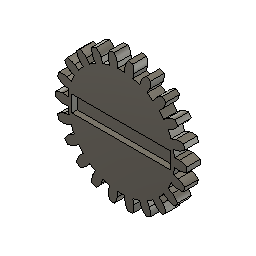
heat_controller (Autodesk Fusion 360 archive; units mm, degrees)
design "gear"
Autodesk Fusion 360 part; units mm, degrees
(part 1 of 8)
sketch "Sketch1" plane through (0, 0, 0) normal (0, 0, 1) x (1, 0, 0) in component "Component"
  spline S0 degree 5 poles (21.2374, -1.6373) (21.2376, -1.6373) (21.2379, -1.6374) (21.2384, -1.6374) (21.2392, -1.6374) (21.2403, -1.6375) (21.2417, -1.6376) (21.2433, -1.6377) (21.245, -1.6378) (21.2469, -1.6378) (21.249, -1.6379) (21.2512, -1.638) (21.2537, -1.6381) (21.2562, -1.6382) (21.259, -1.6383) (21.2619, -1.6384) (21.265, -1.6385) (21.2682, -1.6385) (21.2715, -1.6386) (21.2751, -1.6387) (21.2787, -1.6387) (21.2825, -1.6388) (21.2865, -1.6388) (21.2906, -1.6388) (21.2948, -1.6389) (21.2991, -1.6389) (21.3036, -1.6389) (21.3083, -1.6388) (21.313, -1.6388) (21.3179, -1.6388) (21.3229, -1.6387) (21.3281, -1.6386) (21.3334, -1.6385) (21.3387, -1.6384) (21.3443, -1.6383) (21.3499, -1.6382) (21.3556, -1.638) (21.3615, -1.6378) (21.3675, -1.6376) (21.3736, -1.6374) (21.3798, -1.6372) (21.3861, -1.6369) (21.3925, -1.6367) (21.399, -1.6364) (21.4057, -1.636) (21.4124, -1.6357) (21.4193, -1.6353) (21.4262, -1.6349) (21.4333, -1.6345) (21.4405, -1.6341) (21.4477, -1.6336) (21.4551, -1.6332) (21.4625, -1.6327) (21.4701, -1.6321) (21.4778, -1.6316) (21.4855, -1.631) (21.4934, -1.6304) (21.5013, -1.6298) (21.5093, -1.6291) (21.5174, -1.6284) (21.5257, -1.6277) (21.534, -1.6269) (21.5423, -1.6262) (21.5508, -1.6254) (21.5594, -1.6245) (21.568, -1.6237) (21.5768, -1.6228) (21.5856, -1.6219) (21.5945, -1.621) (21.6035, -1.62) (21.6126, -1.619) (21.6217, -1.6179) (21.631, -1.6169) (21.6403, -1.6158) (21.6497, -1.6147) (21.6592, -1.6135) (21.6687, -1.6123) (21.6783, -1.6111) (21.688, -1.6098) (21.6978, -1.6086) (21.7077, -1.6072) (21.7176, -1.6059) (21.7276, -1.6045) (21.7377, -1.6031) (21.7479, -1.6017) (21.7581, -1.6002) (21.7684, -1.5987) (21.7788, -1.5971) (21.7892, -1.5955) (21.7997, -1.5939) (21.8103, -1.5923) (21.821, -1.5906) (21.8317, -1.5889) (21.8425, -1.5871) (21.8533, -1.5853) (21.8642, -1.5835) (21.8752, -1.5816) (21.8863, -1.5797) (21.8974, -1.5778) (21.9086, -1.5758) (21.9198, -1.5738) (21.9311, -1.5718) (21.9425, -1.5697) (21.9539, -1.5676) (21.9654, -1.5655) (21.977, -1.5633) (21.9886, -1.5611) (22.0003, -1.5588) (22.012, -1.5565) (22.0238, -1.5542) (22.0357, -1.5518) (22.0476, -1.5494) (22.0596, -1.547) (22.0716, -1.5445) (22.0837, -1.542) (22.0958, -1.5394) (22.108, -1.5368) (22.1203, -1.5342) (22.1326, -1.5315) (22.145, -1.5288) (22.1574, -1.5261) (22.1699, -1.5233) (22.1824, -1.5205) (22.195, -1.5176) (22.2077, -1.5147) (22.2204, -1.5118) (22.2331, -1.5088) (22.2459, -1.5058) (22.2588, -1.5027) (22.2717, -1.4996) (22.2846, -1.4965) (22.2976, -1.4933) (22.3107, -1.4901) (22.3238, -1.4868) (22.3369, -1.4835) (22.3501, -1.4802) (22.3634, -1.4768) (22.3767, -1.4734) (22.39, -1.4699) (22.4034, -1.4664) (22.4169, -1.4629) (22.4304, -1.4593) (22.4439, -1.4557) (22.4575, -1.452) (22.4711, -1.4483) (22.4848, -1.4446) (22.4985, -1.4408) (22.5123, -1.437) (22.5261, -1.4331) (22.5399, -1.4292) (22.5538, -1.4253) (22.5678, -1.4213) (22.5818, -1.4172) (22.5958, -1.4132) (22.6099, -1.4091) (22.624, -1.4049) (22.6381, -1.4007) (22.6523, -1.3965) (22.6666, -1.3922) (22.6809, -1.3879) (22.6952, -1.3835) (22.7095, -1.3791) (22.7239, -1.3747) (22.7384, -1.3702) (22.7529, -1.3656) (22.7674, -1.3611) (22.7819, -1.3564) (22.7965, -1.3518) (22.8112, -1.3471) (22.8259, -1.3423) (22.8406, -1.3376) (22.8553, -1.3327) (22.8701, -1.3279) (22.8849, -1.3229) (22.8998, -1.318) (22.9147, -1.313) (22.9297, -1.3079) (22.9446, -1.3029) (22.9596, -1.2977) (22.9747, -1.2926) (22.9898, -1.2874) (23.0049, -1.2821) (23.02, -1.2768) (23.0352, -1.2715) (23.0504, -1.2661) (23.0657, -1.2606) (23.081, -1.2552) (23.0963, -1.2496) (23.1116, -1.2441) (23.127, -1.2385) (23.1425, -1.2328) (23.1579, -1.2271) (23.1734, -1.2214) (23.1889, -1.2156) (23.2045, -1.2098) (23.22, -1.204) (23.2356, -1.198) (23.2513, -1.1921) (23.267, -1.1861) (23.2827, -1.1801) (23.2984, -1.174) (23.3142, -1.1678) (23.33, -1.1617) (23.3458, -1.1555) (23.3617, -1.1492) (23.3775, -1.1429) (23.3934, -1.1366) (23.4094, -1.1302) (23.4254, -1.1237) (23.4414, -1.1172) (23.4574, -1.1107) (23.4734, -1.1042) (23.4895, -1.0975) (23.5056, -1.0909) (23.5218, -1.0842) (23.5379, -1.0774) (23.5541, -1.0707) (23.5704, -1.0638) (23.5866, -1.0569) (23.6029, -1.05) (23.6192, -1.0431) (23.6355, -1.036) (23.6518, -1.029) (23.6682, -1.0219) (23.6846, -1.0147) (23.701, -1.0075) (23.7175, -1.0003) (23.734, -0.993) (23.7505, -0.9857) (23.767, -0.9783) (23.7835, -0.9709) (23.8001, -0.9635) (23.8167, -0.956) (23.8333, -0.9484) (23.85, -0.9408) (23.8666, -0.9332) (23.8833, -0.9255) (23.9, -0.9178) (23.9168, -0.91) (23.9335, -0.9022) (23.9503, -0.8943) (23.9637, -0.888) (23.9738, -0.8833) (23.9806, -0.8801) (23.9839, -0.8785) knots 0 0 0 0 0 0 0.00416667 0.00833333 0.0125 0.01666667 0.02083333 0.025 0.02916667 0.03333333 0.0375 0.04166667 0.04583333 0.05 0.05416667 0.05833333 0.0625 0.06666667 0.07083333 0.075 0.07916667 0.08333333 0.0875 0.09166667 0.09583333 0.1 0.10416667 0.10833333 0.1125 0.11666667 0.12083333 0.125 0.12916667 0.13333333 0.1375 0.14166667 0.14583333 0.15 0.15416667 0.15833333 0.1625 0.16666667 0.17083333 0.175 0.17916667 0.18333333 0.1875 0.19166667 0.19583333 0.2 0.20416667 0.20833333 0.2125 0.21666667 0.22083333 0.225 0.22916667 0.23333333 0.2375 0.24166667 0.24583333 0.25 0.25416667 0.25833333 0.2625 0.26666667 0.27083333 0.275 0.27916667 0.28333333 0.2875 0.29166667 0.29583333 0.3 0.30416667 0.30833333 0.3125 0.31666667 0.32083333 0.325 0.32916667 0.33333333 0.3375 0.34166667 0.34583333 0.35 0.35416667 0.35833333 0.3625 0.36666667 0.37083333 0.375 0.37916667 0.38333333 0.3875 0.39166667 0.39583333 0.4 0.40416667 0.40833333 0.4125 0.41666667 0.42083333 0.425 0.42916667 0.43333333 0.4375 0.44166667 0.44583333 0.45 0.45416667 0.45833333 0.4625 0.46666667 0.47083333 0.475 0.47916667 0.48333333 0.4875 0.49166667 0.49583333 0.5 0.50416667 0.50833333 0.5125 0.51666667 0.52083333 0.525 0.52916667 0.53333333 0.5375 0.54166667 0.54583333 0.55 0.55416667 0.55833333 0.5625 0.56666667 0.57083333 0.575 0.57916667 0.58333333 0.5875 0.59166667 0.59583333 0.6 0.60416667 0.60833333 0.6125 0.61666667 0.62083333 0.625 0.62916667 0.63333333 0.6375 0.64166667 0.64583333 0.65 0.65416667 0.65833333 0.6625 0.66666667 0.67083333 0.675 0.67916667 0.68333333 0.6875 0.69166667 0.69583333 0.7 0.70416667 0.70833333 0.7125 0.71666667 0.72083333 0.725 0.72916667 0.73333333 0.7375 0.74166667 0.74583333 0.75 0.75416667 0.75833333 0.7625 0.76666667 0.77083333 0.775 0.77916667 0.78333333 0.7875 0.79166667 0.79583333 0.8 0.80416667 0.80833333 0.8125 0.81666667 0.82083333 0.825 0.82916667 0.83333333 0.8375 0.84166667 0.84583333 0.85 0.85416667 0.85833333 0.8625 0.86666667 0.87083333 0.875 0.87916667 0.88333333 0.8875 0.89166667 0.89583333 0.9 0.90416667 0.90833333 0.9125 0.91666667 0.92083333 0.925 0.92916667 0.93333333 0.9375 0.94166667 0.94583333 0.95 0.95416667 0.95833333 0.9625 0.96666667 0.97083333 0.975 0.97916667 0.98333333 0.9875 0.99166667 0.99583333 1 1 1 1 1 1
  spline S1 degree 5 poles (21.2374, 1.6373) (21.2376, 1.6373) (21.2379, 1.6374) (21.2384, 1.6374) (21.2392, 1.6374) (21.2403, 1.6375) (21.2417, 1.6376) (21.2433, 1.6377) (21.245, 1.6378) (21.2469, 1.6378) (21.249, 1.6379) (21.2512, 1.638) (21.2537, 1.6381) (21.2562, 1.6382) (21.259, 1.6383) (21.2619, 1.6384) (21.265, 1.6385) (21.2682, 1.6385) (21.2715, 1.6386) (21.2751, 1.6387) (21.2787, 1.6387) (21.2825, 1.6388) (21.2865, 1.6388) (21.2906, 1.6388) (21.2948, 1.6389) (21.2991, 1.6389) (21.3036, 1.6389) (21.3083, 1.6388) (21.313, 1.6388) (21.3179, 1.6388) (21.3229, 1.6387) (21.3281, 1.6386) (21.3334, 1.6385) (21.3387, 1.6384) (21.3443, 1.6383) (21.3499, 1.6382) (21.3556, 1.638) (21.3615, 1.6378) (21.3675, 1.6376) (21.3736, 1.6374) (21.3798, 1.6372) (21.3861, 1.6369) (21.3925, 1.6367) (21.399, 1.6364) (21.4057, 1.636) (21.4124, 1.6357) (21.4193, 1.6353) (21.4262, 1.6349) (21.4333, 1.6345) (21.4405, 1.6341) (21.4477, 1.6336) (21.4551, 1.6332) (21.4625, 1.6327) (21.4701, 1.6321) (21.4778, 1.6316) (21.4855, 1.631) (21.4934, 1.6304) (21.5013, 1.6298) (21.5093, 1.6291) (21.5174, 1.6284) (21.5257, 1.6277) (21.534, 1.6269) (21.5423, 1.6262) (21.5508, 1.6254) (21.5594, 1.6245) (21.568, 1.6237) (21.5768, 1.6228) (21.5856, 1.6219) (21.5945, 1.621) (21.6035, 1.62) (21.6126, 1.619) (21.6217, 1.6179) (21.631, 1.6169) (21.6403, 1.6158) (21.6497, 1.6147) (21.6592, 1.6135) (21.6687, 1.6123) (21.6783, 1.6111) (21.688, 1.6098) (21.6978, 1.6086) (21.7077, 1.6072) (21.7176, 1.6059) (21.7276, 1.6045) (21.7377, 1.6031) (21.7479, 1.6017) (21.7581, 1.6002) (21.7684, 1.5987) (21.7788, 1.5971) (21.7892, 1.5955) (21.7997, 1.5939) (21.8103, 1.5923) (21.821, 1.5906) (21.8317, 1.5889) (21.8425, 1.5871) (21.8533, 1.5853) (21.8642, 1.5835) (21.8752, 1.5816) (21.8863, 1.5797) (21.8974, 1.5778) (21.9086, 1.5758) (21.9198, 1.5738) (21.9311, 1.5718) (21.9425, 1.5697) (21.9539, 1.5676) (21.9654, 1.5655) (21.977, 1.5633) (21.9886, 1.5611) (22.0003, 1.5588) (22.012, 1.5565) (22.0238, 1.5542) (22.0357, 1.5518) (22.0476, 1.5494) (22.0596, 1.547) (22.0716, 1.5445) (22.0837, 1.542) (22.0958, 1.5394) (22.108, 1.5368) (22.1203, 1.5342) (22.1326, 1.5315) (22.145, 1.5288) (22.1574, 1.5261) (22.1699, 1.5233) (22.1824, 1.5205) (22.195, 1.5176) (22.2077, 1.5147) (22.2204, 1.5118) (22.2331, 1.5088) (22.2459, 1.5058) (22.2588, 1.5027) (22.2717, 1.4996) (22.2846, 1.4965) (22.2976, 1.4933) (22.3107, 1.4901) (22.3238, 1.4868) (22.3369, 1.4835) (22.3501, 1.4802) (22.3634, 1.4768) (22.3767, 1.4734) (22.39, 1.4699) (22.4034, 1.4664) (22.4169, 1.4629) (22.4304, 1.4593) (22.4439, 1.4557) (22.4575, 1.452) (22.4711, 1.4483) (22.4848, 1.4446) (22.4985, 1.4408) (22.5123, 1.437) (22.5261, 1.4331) (22.5399, 1.4292) (22.5538, 1.4253) (22.5678, 1.4213) (22.5818, 1.4172) (22.5958, 1.4132) (22.6099, 1.4091) (22.624, 1.4049) (22.6381, 1.4007) (22.6523, 1.3965) (22.6666, 1.3922) (22.6809, 1.3879) (22.6952, 1.3835) (22.7095, 1.3791) (22.7239, 1.3747) (22.7384, 1.3702) (22.7529, 1.3656) (22.7674, 1.3611) (22.7819, 1.3564) (22.7965, 1.3518) (22.8112, 1.3471) (22.8259, 1.3423) (22.8406, 1.3376) (22.8553, 1.3327) (22.8701, 1.3279) (22.8849, 1.3229) (22.8998, 1.318) (22.9147, 1.313) (22.9297, 1.3079) (22.9446, 1.3029) (22.9596, 1.2977) (22.9747, 1.2926) (22.9898, 1.2874) (23.0049, 1.2821) (23.02, 1.2768) (23.0352, 1.2715) (23.0504, 1.2661) (23.0657, 1.2606) (23.081, 1.2552) (23.0963, 1.2496) (23.1116, 1.2441) (23.127, 1.2385) (23.1425, 1.2328) (23.1579, 1.2271) (23.1734, 1.2214) (23.1889, 1.2156) (23.2045, 1.2098) (23.22, 1.204) (23.2356, 1.198) (23.2513, 1.1921) (23.267, 1.1861) (23.2827, 1.1801) (23.2984, 1.174) (23.3142, 1.1678) (23.33, 1.1617) (23.3458, 1.1555) (23.3617, 1.1492) (23.3775, 1.1429) (23.3934, 1.1366) (23.4094, 1.1302) (23.4254, 1.1237) (23.4414, 1.1172) (23.4574, 1.1107) (23.4734, 1.1042) (23.4895, 1.0975) (23.5056, 1.0909) (23.5218, 1.0842) (23.5379, 1.0774) (23.5541, 1.0707) (23.5704, 1.0638) (23.5866, 1.0569) (23.6029, 1.05) (23.6192, 1.0431) (23.6355, 1.036) (23.6518, 1.029) (23.6682, 1.0219) (23.6846, 1.0147) (23.701, 1.0075) (23.7175, 1.0003) (23.734, 0.993) (23.7505, 0.9857) (23.767, 0.9783) (23.7835, 0.9709) (23.8001, 0.9635) (23.8167, 0.956) (23.8333, 0.9484) (23.85, 0.9408) (23.8666, 0.9332) (23.8833, 0.9255) (23.9, 0.9178) (23.9168, 0.91) (23.9335, 0.9022) (23.9503, 0.8943) (23.9637, 0.888) (23.9738, 0.8833) (23.9806, 0.8801) (23.9839, 0.8785) knots 0 0 0 0 0 0 0.00416667 0.00833333 0.0125 0.01666667 0.02083333 0.025 0.02916667 0.03333333 0.0375 0.04166667 0.04583333 0.05 0.05416667 0.05833333 0.0625 0.06666667 0.07083333 0.075 0.07916667 0.08333333 0.0875 0.09166667 0.09583333 0.1 0.10416667 0.10833333 0.1125 0.11666667 0.12083333 0.125 0.12916667 0.13333333 0.1375 0.14166667 0.14583333 0.15 0.15416667 0.15833333 0.1625 0.16666667 0.17083333 0.175 0.17916667 0.18333333 0.1875 0.19166667 0.19583333 0.2 0.20416667 0.20833333 0.2125 0.21666667 0.22083333 0.225 0.22916667 0.23333333 0.2375 0.24166667 0.24583333 0.25 0.25416667 0.25833333 0.2625 0.26666667 0.27083333 0.275 0.27916667 0.28333333 0.2875 0.29166667 0.29583333 0.3 0.30416667 0.30833333 0.3125 0.31666667 0.32083333 0.325 0.32916667 0.33333333 0.3375 0.34166667 0.34583333 0.35 0.35416667 0.35833333 0.3625 0.36666667 0.37083333 0.375 0.37916667 0.38333333 0.3875 0.39166667 0.39583333 0.4 0.40416667 0.40833333 0.4125 0.41666667 0.42083333 0.425 0.42916667 0.43333333 0.4375 0.44166667 0.44583333 0.45 0.45416667 0.45833333 0.4625 0.46666667 0.47083333 0.475 0.47916667 0.48333333 0.4875 0.49166667 0.49583333 0.5 0.50416667 0.50833333 0.5125 0.51666667 0.52083333 0.525 0.52916667 0.53333333 0.5375 0.54166667 0.54583333 0.55 0.55416667 0.55833333 0.5625 0.56666667 0.57083333 0.575 0.57916667 0.58333333 0.5875 0.59166667 0.59583333 0.6 0.60416667 0.60833333 0.6125 0.61666667 0.62083333 0.625 0.62916667 0.63333333 0.6375 0.64166667 0.64583333 0.65 0.65416667 0.65833333 0.6625 0.66666667 0.67083333 0.675 0.67916667 0.68333333 0.6875 0.69166667 0.69583333 0.7 0.70416667 0.70833333 0.7125 0.71666667 0.72083333 0.725 0.72916667 0.73333333 0.7375 0.74166667 0.74583333 0.75 0.75416667 0.75833333 0.7625 0.76666667 0.77083333 0.775 0.77916667 0.78333333 0.7875 0.79166667 0.79583333 0.8 0.80416667 0.80833333 0.8125 0.81666667 0.82083333 0.825 0.82916667 0.83333333 0.8375 0.84166667 0.84583333 0.85 0.85416667 0.85833333 0.8625 0.86666667 0.87083333 0.875 0.87916667 0.88333333 0.8875 0.89166667 0.89583333 0.9 0.90416667 0.90833333 0.9125 0.91666667 0.92083333 0.925 0.92916667 0.93333333 0.9375 0.94166667 0.94583333 0.95 0.95416667 0.95833333 0.9625 0.96666667 0.97083333 0.975 0.97916667 0.98333333 0.9875 0.99166667 0.99583333 1 1 1 1 1 1
  spline S2 degree 5 poles (21.2362, -1.6372) (21.2363, -1.6373) (21.2364, -1.6373) (21.2365, -1.6373) (21.2367, -1.6373) (21.2369, -1.6373) (21.2371, -1.6373) (21.2373, -1.6373) (21.2374, -1.6373) (21.2374, -1.6373) knots 0 0 0 0 0 0 0.2 0.4 0.6 0.8 1 1 1 1 1 1
  spline S3 degree 5 poles (21.2362, 1.6372) (21.2363, 1.6373) (21.2364, 1.6373) (21.2365, 1.6373) (21.2367, 1.6373) (21.2369, 1.6373) (21.2371, 1.6373) (21.2373, 1.6373) (21.2374, 1.6373) (21.2374, 1.6373) knots 0 0 0 0 0 0 0.2 0.4 0.6 0.8 1 1 1 1 1 1
  line L0 (0, 0) -> (21.2362, -1.6372)
  line L1 (0, 0) -> (21.2362, 1.6372)
  arc A0 (23.9839, -0.8785) -> (23.9839, 0.8785) centre (0, 0) ccw
  point P0 (21.241, -1.6375)
  point P1 (21.247, -1.6378)
  point P2 (21.2553, -1.6382)
  point P3 (21.2661, -1.6385)
  point P4 (21.2793, -1.6387)
  point P5 (21.2948, -1.6389)
  point P6 (21.3128, -1.6388)
  point P7 (21.3331, -1.6385)
  point P8 (21.3558, -1.638)
  point P9 (21.3809, -1.6371)
  point P10 (21.4084, -1.6359)
  point P11 (21.4383, -1.6342)
  point P12 (21.4705, -1.6321)
  point P13 (21.5051, -1.6294)
  point P14 (21.542, -1.6262)
  point P15 (21.5813, -1.6223)
  point P16 (21.6229, -1.6178)
  point P17 (21.6668, -1.6125)
  point P18 (21.7131, -1.6065)
  point P19 (21.7617, -1.5996)
  point P20 (21.8125, -1.5919)
  point P21 (21.8656, -1.5833)
  point P22 (21.921, -1.5736)
  point P23 (21.9787, -1.563)
  point P24 (22.0385, -1.5512)
  point P25 (22.1006, -1.5384)
  point P26 (22.1649, -1.5244)
  point P27 (22.2314, -1.5092)
  point P28 (22.3, -1.4927)
  point P29 (22.3707, -1.4749)
  point P30 (22.4436, -1.4558)
  point P31 (22.5186, -1.4352)
  point P32 (22.5957, -1.4132)
  point P33 (22.6748, -1.3897)
  point P34 (22.7559, -1.3647)
  point P35 (22.8391, -1.338)
  point P36 (22.9242, -1.3098)
  point P37 (23.0113, -1.2798)
  point P38 (23.1004, -1.2482)
  point P39 (23.1913, -1.2147)
  point P40 (23.2841, -1.1795)
  point P41 (23.3788, -1.1424)
  point P42 (23.4753, -1.1034)
  point P43 (23.5735, -1.0625)
  point P44 (23.6736, -1.0195)
  point P45 (23.7753, -0.9746)
  point P46 (23.8788, -0.9276)
  point P47 (21.241, 1.6375)
  point P48 (21.247, 1.6378)
  point P49 (21.2553, 1.6382)
  point P50 (21.2661, 1.6385)
  point P51 (21.2793, 1.6387)
  point P52 (21.2948, 1.6389)
  point P53 (21.3128, 1.6388)
  point P54 (21.3331, 1.6385)
  point P55 (21.3558, 1.638)
  point P56 (21.3809, 1.6371)
  point P57 (21.4084, 1.6359)
  point P58 (21.4383, 1.6342)
  point P59 (21.4705, 1.6321)
  point P60 (21.5051, 1.6294)
  point P61 (21.542, 1.6262)
  point P62 (21.5813, 1.6223)
  point P63 (21.6229, 1.6178)
  point P64 (21.6668, 1.6125)
  point P65 (21.7131, 1.6065)
  point P66 (21.7617, 1.5996)
  point P67 (21.8125, 1.5919)
  point P68 (21.8656, 1.5833)
  point P69 (21.921, 1.5736)
  point P70 (21.9787, 1.563)
  point P71 (22.0385, 1.5512)
  point P72 (22.1006, 1.5384)
  point P73 (22.1649, 1.5244)
  point P74 (22.2314, 1.5092)
  point P75 (22.3, 1.4927)
  point P76 (22.3707, 1.4749)
  point P77 (22.4436, 1.4558)
  point P78 (22.5186, 1.4352)
  point P79 (22.5957, 1.4132)
  point P80 (22.6748, 1.3897)
  point P81 (22.7559, 1.3647)
  point P82 (22.8391, 1.338)
  point P83 (22.9242, 1.3098)
  point P84 (23.0113, 1.2798)
  point P85 (23.1004, 1.2482)
  point P86 (23.1913, 1.2147)
  point P87 (23.2841, 1.1795)
  point P88 (23.3788, 1.1424)
  point P89 (23.4753, 1.1034)
  point P90 (23.5735, 1.0625)
  point P91 (23.6736, 1.0195)
  point P92 (23.7753, 0.9746)
  point P93 (23.8788, 0.9276)
sketch "Sketch2" plane through (0, 0, 0) normal (0, 0, 1) x (1, 0, 0) in component "Component"
  circle A0 centre (0, 0) radius 19.5
extrude "Extrude1" add sketch "Sketch2" along normal blind 10 makes body 1 in component "Component"
extrude "Extrude2" add sketch "Sketch1" along normal blind 10 separate body makes body 2 in component "Component"
pattern_circular "C-Pattern1" count 22 over 360 about axis through (0, 0, 1.75) along (0, 0, 1) of "Extrude2" makes body 3 at (6.6386, 2.5181, 3.3333) makes body 4 at (6.2504, 3.3681, 3.3333) makes body 5 at (5.0483, 4.9926, 3.3333) makes body 6 at (2.4443, 6.6661, 3.3333) makes body 7 at (1.5477, 6.9294, 3.3333) makes body 8 at (-0.4672, 7.0848, 3.3333) makes body 9 at (-2.4443, 6.6661, 3.3333) makes body 10 at (-5.0483, 4.9926, 3.3333) makes body 11 at (-5.6603, 4.2864, 3.3333) makes body 12 at (-6.6386, 2.5181, 3.3333) makes body 13 at (-7.0791, 0.5458, 6.6667) makes body 14 at (-6.6386, -2.5181, 3.3333) makes body 15 at (-6.2504, -3.3681, 3.3333) makes body 16 at (-5.0483, -4.9926, 3.3333) makes body 17 at (-2.4443, -6.6661, 3.3333) makes body 18 at (-1.5477, -6.9294, 3.3333) makes body 19 at (1.5477, -6.9294, 3.3333) makes body 20 at (2.4443, -6.6661, 3.3333) makes body 21 at (5.0483, -4.9926, 3.3333) makes body 22 at (5.6603, -4.2864, 6.6667) makes body 23 at (6.6386, -2.5181, 3.3333) in component "Component"
combine "Combine1" operation add target body 1 tool bodies 2 3 4 5 6 7 8 9 10 11 12 13 14 15 16 17 18 19 20 21 22 23 in component "Component"
sketch "Sketch3" plane through (0, 0, 0) normal (0, 0, 1) x (1, 0, 0) in component "Component"
  line L0 (0, 0) -> (50.7993, 0) construction
  line L1 (50.7993, 0) -> (50.7993, 3) construction
  line L2 (50.7993, 3) -> (0, 3) construction
  line L3 (0, 3) -> (0, 0) construction
  constraint perpendicular L0 L1
  constraint parallel L0 L2
  constraint parallel L1 L3
sketch "Sketch1 (2)" plane through (0, 0, 10) normal (0, 0, 1) x (1, 0, 0)
  arc A0 (19.0771, -4.0393) -> (19.4423, -1.4989) centre (0, 0) ccw
  line L0 (19.4423, -1.4989) -> (21.2362, -1.6372)
  line L1 (21.2362, -1.6372) -> (21.2374, -1.6373)
  spline S0 degree 5 poles (21.2374, -1.6373) (21.2376, -1.6373) (21.2379, -1.6374) (21.2384, -1.6374) (21.2392, -1.6374) (21.2403, -1.6375) (21.2417, -1.6376) (21.2433, -1.6377) (21.245, -1.6378) (21.2469, -1.6378) (21.249, -1.6379) (21.2512, -1.638) (21.2537, -1.6381) (21.2562, -1.6382) (21.259, -1.6383) (21.2619, -1.6384) (21.265, -1.6385) (21.2682, -1.6385) (21.2715, -1.6386) (21.2751, -1.6387) (21.2787, -1.6387) (21.2825, -1.6388) (21.2865, -1.6388) (21.2906, -1.6388) (21.2948, -1.6389) (21.2991, -1.6389) (21.3036, -1.6389) (21.3083, -1.6388) (21.313, -1.6388) (21.3179, -1.6388) (21.3229, -1.6387) (21.3281, -1.6386) (21.3334, -1.6385) (21.3387, -1.6384) (21.3443, -1.6383) (21.3499, -1.6382) (21.3556, -1.638) (21.3615, -1.6378) (21.3675, -1.6376) (21.3736, -1.6374) (21.3798, -1.6372) (21.3861, -1.6369) (21.3925, -1.6367) (21.399, -1.6364) (21.4057, -1.636) (21.4124, -1.6357) (21.4193, -1.6353) (21.4262, -1.6349) (21.4333, -1.6345) (21.4405, -1.6341) (21.4477, -1.6336) (21.4551, -1.6332) (21.4625, -1.6327) (21.4701, -1.6321) (21.4778, -1.6316) (21.4855, -1.631) (21.4934, -1.6304) (21.5013, -1.6298) (21.5093, -1.6291) (21.5174, -1.6284) (21.5257, -1.6277) (21.534, -1.6269) (21.5423, -1.6262) (21.5508, -1.6254) (21.5594, -1.6245) (21.568, -1.6237) (21.5768, -1.6228) (21.5856, -1.6219) (21.5945, -1.621) (21.6035, -1.62) (21.6126, -1.619) (21.6217, -1.6179) (21.631, -1.6169) (21.6403, -1.6158) (21.6497, -1.6147) (21.6592, -1.6135) (21.6687, -1.6123) (21.6783, -1.6111) (21.688, -1.6098) (21.6978, -1.6086) (21.7077, -1.6072) (21.7176, -1.6059) (21.7276, -1.6045) (21.7377, -1.6031) (21.7479, -1.6017) (21.7581, -1.6002) (21.7684, -1.5987) (21.7788, -1.5971) (21.7892, -1.5955) (21.7997, -1.5939) (21.8103, -1.5923) (21.821, -1.5906) (21.8317, -1.5889) (21.8425, -1.5871) (21.8533, -1.5853) (21.8642, -1.5835) (21.8752, -1.5816) (21.8863, -1.5797) (21.8974, -1.5778) (21.9086, -1.5758) (21.9198, -1.5738) (21.9311, -1.5718) (21.9425, -1.5697) (21.9539, -1.5676) (21.9654, -1.5655) (21.977, -1.5633) (21.9886, -1.5611) (22.0003, -1.5588) (22.012, -1.5565) (22.0238, -1.5542) (22.0357, -1.5518) (22.0476, -1.5494) (22.0596, -1.547) (22.0716, -1.5445) (22.0837, -1.542) (22.0958, -1.5394) (22.108, -1.5368) (22.1203, -1.5342) (22.1326, -1.5315) (22.145, -1.5288) (22.1574, -1.5261) (22.1699, -1.5233) (22.1824, -1.5205) (22.195, -1.5176) (22.2077, -1.5147) (22.2204, -1.5118) (22.2331, -1.5088) (22.2459, -1.5058) (22.2588, -1.5027) (22.2717, -1.4996) (22.2846, -1.4965) (22.2976, -1.4933) (22.3107, -1.4901) (22.3238, -1.4868) (22.3369, -1.4835) (22.3501, -1.4802) (22.3634, -1.4768) (22.3767, -1.4734) (22.39, -1.4699) (22.4034, -1.4664) (22.4169, -1.4629) (22.4304, -1.4593) (22.4439, -1.4557) (22.4575, -1.452) (22.4711, -1.4483) (22.4848, -1.4446) (22.4985, -1.4408) (22.5123, -1.437) (22.5261, -1.4331) (22.5399, -1.4292) (22.5538, -1.4253) (22.5678, -1.4213) (22.5818, -1.4172) (22.5958, -1.4132) (22.6099, -1.4091) (22.624, -1.4049) (22.6381, -1.4007) (22.6523, -1.3965) (22.6666, -1.3922) (22.6809, -1.3879) (22.6952, -1.3835) (22.7095, -1.3791) (22.7239, -1.3747) (22.7384, -1.3702) (22.7529, -1.3656) (22.7674, -1.3611) (22.7819, -1.3564) (22.7965, -1.3518) (22.8112, -1.3471) (22.8259, -1.3423) (22.8406, -1.3376) (22.8553, -1.3327) (22.8701, -1.3279) (22.8849, -1.3229) (22.8998, -1.318) (22.9147, -1.313) (22.9297, -1.3079) (22.9446, -1.3029) (22.9596, -1.2977) (22.9747, -1.2926) (22.9898, -1.2874) (23.0049, -1.2821) (23.02, -1.2768) (23.0352, -1.2715) (23.0504, -1.2661) (23.0657, -1.2606) (23.081, -1.2552) (23.0963, -1.2496) (23.1116, -1.2441) (23.127, -1.2385) (23.1425, -1.2328) (23.1579, -1.2271) (23.1734, -1.2214) (23.1889, -1.2156) (23.2045, -1.2098) (23.22, -1.204) (23.2356, -1.198) (23.2513, -1.1921) (23.267, -1.1861) (23.2827, -1.1801) (23.2984, -1.174) (23.3142, -1.1678) (23.33, -1.1617) (23.3458, -1.1555) (23.3617, -1.1492) (23.3775, -1.1429) (23.3934, -1.1366) (23.4094, -1.1302) (23.4254, -1.1237) (23.4414, -1.1172) (23.4574, -1.1107) (23.4734, -1.1042) (23.4895, -1.0975) (23.5056, -1.0909) (23.5218, -1.0842) (23.5379, -1.0774) (23.5541, -1.0707) (23.5704, -1.0638) (23.5866, -1.0569) (23.6029, -1.05) (23.6192, -1.0431) (23.6355, -1.036) (23.6518, -1.029) (23.6682, -1.0219) (23.6846, -1.0147) (23.701, -1.0075) (23.7175, -1.0003) (23.734, -0.993) (23.7505, -0.9857) (23.767, -0.9783) (23.7835, -0.9709) (23.8001, -0.9635) (23.8167, -0.956) (23.8333, -0.9484) (23.85, -0.9408) (23.8666, -0.9332) (23.8833, -0.9255) (23.9, -0.9178) (23.9168, -0.91) (23.9335, -0.9022) (23.9503, -0.8943) (23.9637, -0.888) (23.9738, -0.8833) (23.9806, -0.8801) (23.9839, -0.8785) knots 0 0 0 0 0 0 0.00416667 0.00833333 0.0125 0.01666667 0.02083333 0.025 0.02916667 0.03333333 0.0375 0.04166667 0.04583333 0.05 0.05416667 0.05833333 0.0625 0.06666667 0.07083333 0.075 0.07916667 0.08333333 0.0875 0.09166667 0.09583333 0.1 0.10416667 0.10833333 0.1125 0.11666667 0.12083333 0.125 0.12916667 0.13333333 0.1375 0.14166667 0.14583333 0.15 0.15416667 0.15833333 0.1625 0.16666667 0.17083333 0.175 0.17916667 0.18333333 0.1875 0.19166667 0.19583333 0.2 0.20416667 0.20833333 0.2125 0.21666667 0.22083333 0.225 0.22916667 0.23333333 0.2375 0.24166667 0.24583333 0.25 0.25416667 0.25833333 0.2625 0.26666667 0.27083333 0.275 0.27916667 0.28333333 0.2875 0.29166667 0.29583333 0.3 0.30416667 0.30833333 0.3125 0.31666667 0.32083333 0.325 0.32916667 0.33333333 0.3375 0.34166667 0.34583333 0.35 0.35416667 0.35833333 0.3625 0.36666667 0.37083333 0.375 0.37916667 0.38333333 0.3875 0.39166667 0.39583333 0.4 0.40416667 0.40833333 0.4125 0.41666667 0.42083333 0.425 0.42916667 0.43333333 0.4375 0.44166667 0.44583333 0.45 0.45416667 0.45833333 0.4625 0.46666667 0.47083333 0.475 0.47916667 0.48333333 0.4875 0.49166667 0.49583333 0.5 0.50416667 0.50833333 0.5125 0.51666667 0.52083333 0.525 0.52916667 0.53333333 0.5375 0.54166667 0.54583333 0.55 0.55416667 0.55833333 0.5625 0.56666667 0.57083333 0.575 0.57916667 0.58333333 0.5875 0.59166667 0.59583333 0.6 0.60416667 0.60833333 0.6125 0.61666667 0.62083333 0.625 0.62916667 0.63333333 0.6375 0.64166667 0.64583333 0.65 0.65416667 0.65833333 0.6625 0.66666667 0.67083333 0.675 0.67916667 0.68333333 0.6875 0.69166667 0.69583333 0.7 0.70416667 0.70833333 0.7125 0.71666667 0.72083333 0.725 0.72916667 0.73333333 0.7375 0.74166667 0.74583333 0.75 0.75416667 0.75833333 0.7625 0.76666667 0.77083333 0.775 0.77916667 0.78333333 0.7875 0.79166667 0.79583333 0.8 0.80416667 0.80833333 0.8125 0.81666667 0.82083333 0.825 0.82916667 0.83333333 0.8375 0.84166667 0.84583333 0.85 0.85416667 0.85833333 0.8625 0.86666667 0.87083333 0.875 0.87916667 0.88333333 0.8875 0.89166667 0.89583333 0.9 0.90416667 0.90833333 0.9125 0.91666667 0.92083333 0.925 0.92916667 0.93333333 0.9375 0.94166667 0.94583333 0.95 0.95416667 0.95833333 0.9625 0.96666667 0.97083333 0.975 0.97916667 0.98333333 0.9875 0.99166667 0.99583333 1 1 1 1 1 1
  arc A1 (23.9839, -0.8785) -> (23.9839, 0.8785) centre (0, 0) ccw
  spline S1 degree 5 poles (23.9839, 0.8785) (23.9806, 0.8801) (23.9738, 0.8833) (23.9637, 0.888) (23.9503, 0.8943) (23.9335, 0.9022) (23.9168, 0.91) (23.9, 0.9178) (23.8833, 0.9255) (23.8666, 0.9332) (23.85, 0.9408) (23.8333, 0.9484) (23.8167, 0.956) (23.8001, 0.9635) (23.7835, 0.9709) (23.767, 0.9783) (23.7505, 0.9857) (23.734, 0.993) (23.7175, 1.0003) (23.701, 1.0075) (23.6846, 1.0147) (23.6682, 1.0219) (23.6518, 1.029) (23.6355, 1.036) (23.6192, 1.0431) (23.6029, 1.05) (23.5866, 1.0569) (23.5704, 1.0638) (23.5541, 1.0707) (23.5379, 1.0774) (23.5218, 1.0842) (23.5056, 1.0909) (23.4895, 1.0975) (23.4734, 1.1042) (23.4574, 1.1107) (23.4414, 1.1172) (23.4254, 1.1237) (23.4094, 1.1302) (23.3934, 1.1366) (23.3775, 1.1429) (23.3617, 1.1492) (23.3458, 1.1555) (23.33, 1.1617) (23.3142, 1.1678) (23.2984, 1.174) (23.2827, 1.1801) (23.267, 1.1861) (23.2513, 1.1921) (23.2356, 1.198) (23.22, 1.204) (23.2045, 1.2098) (23.1889, 1.2156) (23.1734, 1.2214) (23.1579, 1.2271) (23.1425, 1.2328) (23.127, 1.2385) (23.1116, 1.2441) (23.0963, 1.2496) (23.081, 1.2552) (23.0657, 1.2606) (23.0504, 1.2661) (23.0352, 1.2715) (23.02, 1.2768) (23.0049, 1.2821) (22.9898, 1.2874) (22.9747, 1.2926) (22.9596, 1.2977) (22.9446, 1.3029) (22.9297, 1.3079) (22.9147, 1.313) (22.8998, 1.318) (22.8849, 1.3229) (22.8701, 1.3279) (22.8553, 1.3327) (22.8406, 1.3376) (22.8259, 1.3423) (22.8112, 1.3471) (22.7965, 1.3518) (22.7819, 1.3564) (22.7674, 1.3611) (22.7529, 1.3656) (22.7384, 1.3702) (22.7239, 1.3747) (22.7095, 1.3791) (22.6952, 1.3835) (22.6809, 1.3879) (22.6666, 1.3922) (22.6523, 1.3965) (22.6381, 1.4007) (22.624, 1.4049) (22.6099, 1.4091) (22.5958, 1.4132) (22.5818, 1.4172) (22.5678, 1.4213) (22.5538, 1.4253) (22.5399, 1.4292) (22.5261, 1.4331) (22.5123, 1.437) (22.4985, 1.4408) (22.4848, 1.4446) (22.4711, 1.4483) (22.4575, 1.452) (22.4439, 1.4557) (22.4304, 1.4593) (22.4169, 1.4629) (22.4034, 1.4664) (22.39, 1.4699) (22.3767, 1.4734) (22.3634, 1.4768) (22.3501, 1.4802) (22.3369, 1.4835) (22.3238, 1.4868) (22.3107, 1.4901) (22.2976, 1.4933) (22.2846, 1.4965) (22.2717, 1.4996) (22.2588, 1.5027) (22.2459, 1.5058) (22.2331, 1.5088) (22.2204, 1.5118) (22.2077, 1.5147) (22.195, 1.5176) (22.1824, 1.5205) (22.1699, 1.5233) (22.1574, 1.5261) (22.145, 1.5288) (22.1326, 1.5315) (22.1203, 1.5342) (22.108, 1.5368) (22.0958, 1.5394) (22.0837, 1.542) (22.0716, 1.5445) (22.0596, 1.547) (22.0476, 1.5494) (22.0357, 1.5518) (22.0238, 1.5542) (22.012, 1.5565) (22.0003, 1.5588) (21.9886, 1.5611) (21.977, 1.5633) (21.9654, 1.5655) (21.9539, 1.5676) (21.9425, 1.5697) (21.9311, 1.5718) (21.9198, 1.5738) (21.9086, 1.5758) (21.8974, 1.5778) (21.8863, 1.5797) (21.8752, 1.5816) (21.8642, 1.5835) (21.8533, 1.5853) (21.8425, 1.5871) (21.8317, 1.5889) (21.821, 1.5906) (21.8103, 1.5923) (21.7997, 1.5939) (21.7892, 1.5955) (21.7788, 1.5971) (21.7684, 1.5987) (21.7581, 1.6002) (21.7479, 1.6017) (21.7377, 1.6031) (21.7276, 1.6045) (21.7176, 1.6059) (21.7077, 1.6072) (21.6978, 1.6086) (21.688, 1.6098) (21.6783, 1.6111) (21.6687, 1.6123) (21.6592, 1.6135) (21.6497, 1.6147) (21.6403, 1.6158) (21.631, 1.6169) (21.6217, 1.6179) (21.6126, 1.619) (21.6035, 1.62) (21.5945, 1.621) (21.5856, 1.6219) (21.5768, 1.6228) (21.568, 1.6237) (21.5594, 1.6245) (21.5508, 1.6254) (21.5423, 1.6262) (21.534, 1.6269) (21.5257, 1.6277) (21.5174, 1.6284) (21.5093, 1.6291) (21.5013, 1.6298) (21.4934, 1.6304) (21.4855, 1.631) (21.4778, 1.6316) (21.4701, 1.6321) (21.4625, 1.6327) (21.4551, 1.6332) (21.4477, 1.6336) (21.4405, 1.6341) (21.4333, 1.6345) (21.4262, 1.6349) (21.4193, 1.6353) (21.4124, 1.6357) (21.4057, 1.636) (21.399, 1.6364) (21.3925, 1.6367) (21.3861, 1.6369) (21.3798, 1.6372) (21.3736, 1.6374) (21.3675, 1.6376) (21.3615, 1.6378) (21.3556, 1.638) (21.3499, 1.6382) (21.3443, 1.6383) (21.3387, 1.6384) (21.3334, 1.6385) (21.3281, 1.6386) (21.3229, 1.6387) (21.3179, 1.6388) (21.313, 1.6388) (21.3083, 1.6388) (21.3036, 1.6389) (21.2991, 1.6389) (21.2948, 1.6389) (21.2906, 1.6388) (21.2865, 1.6388) (21.2825, 1.6388) (21.2787, 1.6387) (21.2751, 1.6387) (21.2715, 1.6386) (21.2682, 1.6385) (21.265, 1.6385) (21.2619, 1.6384) (21.259, 1.6383) (21.2562, 1.6382) (21.2537, 1.6381) (21.2512, 1.638) (21.249, 1.6379) (21.2469, 1.6378) (21.245, 1.6378) (21.2433, 1.6377) (21.2417, 1.6376) (21.2403, 1.6375) (21.2392, 1.6374) (21.2384, 1.6374) (21.2379, 1.6374) (21.2376, 1.6373) (21.2374, 1.6373) knots -1 -1 -1 -1 -1 -1 -0.99583333 -0.99166667 -0.9875 -0.98333333 -0.97916667 -0.975 -0.97083333 -0.96666667 -0.9625 -0.95833333 -0.95416667 -0.95 -0.94583333 -0.94166667 -0.9375 -0.93333333 -0.92916667 -0.925 -0.92083333 -0.91666667 -0.9125 -0.90833333 -0.90416667 -0.9 -0.89583333 -0.89166667 -0.8875 -0.88333333 -0.87916667 -0.875 -0.87083333 -0.86666667 -0.8625 -0.85833333 -0.85416667 -0.85 -0.84583333 -0.84166667 -0.8375 -0.83333333 -0.82916667 -0.825 -0.82083333 -0.81666667 -0.8125 -0.80833333 -0.80416667 -0.8 -0.79583333 -0.79166667 -0.7875 -0.78333333 -0.77916667 -0.775 -0.77083333 -0.76666667 -0.7625 -0.75833333 -0.75416667 -0.75 -0.74583333 -0.74166667 -0.7375 -0.73333333 -0.72916667 -0.725 -0.72083333 -0.71666667 -0.7125 -0.70833333 -0.70416667 -0.7 -0.69583333 -0.69166667 -0.6875 -0.68333333 -0.67916667 -0.675 -0.67083333 -0.66666667 -0.6625 -0.65833333 -0.65416667 -0.65 -0.64583333 -0.64166667 -0.6375 -0.63333333 -0.62916667 -0.625 -0.62083333 -0.61666667 -0.6125 -0.60833333 -0.60416667 -0.6 -0.59583333 -0.59166667 -0.5875 -0.58333333 -0.57916667 -0.575 -0.57083333 -0.56666667 -0.5625 -0.55833333 -0.55416667 -0.55 -0.54583333 -0.54166667 -0.5375 -0.53333333 -0.52916667 -0.525 -0.52083333 -0.51666667 -0.5125 -0.50833333 -0.50416667 -0.5 -0.49583333 -0.49166667 -0.4875 -0.48333333 -0.47916667 -0.475 -0.47083333 -0.46666667 -0.4625 -0.45833333 -0.45416667 -0.45 -0.44583333 -0.44166667 -0.4375 -0.43333333 -0.42916667 -0.425 -0.42083333 -0.41666667 -0.4125 -0.40833333 -0.40416667 -0.4 -0.39583333 -0.39166667 -0.3875 -0.38333333 -0.37916667 -0.375 -0.37083333 -0.36666667 -0.3625 -0.35833333 -0.35416667 -0.35 -0.34583333 -0.34166667 -0.3375 -0.33333333 -0.32916667 -0.325 -0.32083333 -0.31666667 -0.3125 -0.30833333 -0.30416667 -0.3 -0.29583333 -0.29166667 -0.2875 -0.28333333 -0.27916667 -0.275 -0.27083333 -0.26666667 -0.2625 -0.25833333 -0.25416667 -0.25 -0.24583333 -0.24166667 -0.2375 -0.23333333 -0.22916667 -0.225 -0.22083333 -0.21666667 -0.2125 -0.20833333 -0.20416667 -0.2 -0.19583333 -0.19166667 -0.1875 -0.18333333 -0.17916667 -0.175 -0.17083333 -0.16666667 -0.1625 -0.15833333 -0.15416667 -0.15 -0.14583333 -0.14166667 -0.1375 -0.13333333 -0.12916667 -0.125 -0.12083333 -0.11666667 -0.1125 -0.10833333 -0.10416667 -0.1 -0.09583333 -0.09166667 -0.0875 -0.08333333 -0.07916667 -0.075 -0.07083333 -0.06666667 -0.0625 -0.05833333 -0.05416667 -0.05 -0.04583333 -0.04166667 -0.0375 -0.03333333 -0.02916667 -0.025 -0.02083333 -0.01666667 -0.0125 -0.00833333 -0.00416667 0 0 0 0 0 0
  line L2 (21.2374, 1.6373) -> (21.2362, 1.6372)
  line L3 (21.2362, 1.6372) -> (19.4423, 1.4989)
  arc A2 (19.4423, 1.4989) -> (19.0771, 4.0393) centre (0, 0) ccw
  line L4 (19.0771, 4.0393) -> (20.8373, 4.412)
  line L5 (20.8373, 4.412) -> (20.8384, 4.4123)
  spline S2 degree 5 poles (20.8384, 4.4123) (20.8386, 4.4123) (20.8389, 4.4124) (20.8394, 4.4125) (20.8402, 4.4126) (20.8413, 4.4129) (20.8426, 4.4132) (20.8441, 4.4136) (20.8458, 4.414) (20.8477, 4.4144) (20.8497, 4.4149) (20.8519, 4.4155) (20.8543, 4.4161) (20.8568, 4.4167) (20.8594, 4.4174) (20.8622, 4.4181) (20.8652, 4.4189) (20.8683, 4.4198) (20.8715, 4.4206) (20.8749, 4.4216) (20.8785, 4.4226) (20.8821, 4.4236) (20.8859, 4.4247) (20.8899, 4.4258) (20.8939, 4.427) (20.8981, 4.4282) (20.9024, 4.4295) (20.9069, 4.4308) (20.9114, 4.4321) (20.9161, 4.4336) (20.9209, 4.435) (20.9258, 4.4366) (20.9308, 4.4381) (20.936, 4.4398) (20.9412, 4.4414) (20.9466, 4.4431) (20.9521, 4.4449) (20.9576, 4.4467) (20.9633, 4.4486) (20.9691, 4.4505) (20.975, 4.4525) (20.981, 4.4545) (20.9871, 4.4566) (20.9932, 4.4587) (20.9995, 4.4609) (21.0059, 4.4631) (21.0124, 4.4654) (21.0189, 4.4678) (21.0256, 4.4701) (21.0324, 4.4726) (21.0392, 4.4751) (21.0461, 4.4776) (21.0531, 4.4802) (21.0602, 4.4828) (21.0674, 4.4855) (21.0747, 4.4882) (21.0821, 4.491) (21.0895, 4.4939) (21.097, 4.4968) (21.1046, 4.4997) (21.1123, 4.5027) (21.12, 4.5058) (21.1279, 4.5089) (21.1358, 4.512) (21.1438, 4.5152) (21.1518, 4.5185) (21.16, 4.5218) (21.1682, 4.5252) (21.1765, 4.5286) (21.1848, 4.5321) (21.1932, 4.5356) (21.2017, 4.5391) (21.2103, 4.5428) (21.2189, 4.5464) (21.2276, 4.5502) (21.2364, 4.5539) (21.2452, 4.5578) (21.2541, 4.5617) (21.2631, 4.5656) (21.2721, 4.5696) (21.2812, 4.5736) (21.2903, 4.5777) (21.2996, 4.5819) (21.3088, 4.5861) (21.3182, 4.5903) (21.3276, 4.5946) (21.337, 4.599) (21.3465, 4.6034) (21.3561, 4.6078) (21.3657, 4.6123) (21.3754, 4.6169) (21.3852, 4.6215) (21.395, 4.6262) (21.4048, 4.6309) (21.4147, 4.6357) (21.4247, 4.6405) (21.4347, 4.6454) (21.4448, 4.6503) (21.4549, 4.6553) (21.4651, 4.6603) (21.4753, 4.6654) (21.4856, 4.6706) (21.4959, 4.6758) (21.5063, 4.681) (21.5167, 4.6863) (21.5272, 4.6917) (21.5377, 4.6971) (21.5483, 4.7025) (21.5589, 4.708) (21.5696, 4.7136) (21.5803, 4.7192) (21.591, 4.7249) (21.6018, 4.7306) (21.6127, 4.7364) (21.6236, 4.7422) (21.6345, 4.748) (21.6455, 4.754) (21.6565, 4.76) (21.6676, 4.766) (21.6787, 4.7721) (21.6898, 4.7782) (21.701, 4.7844) (21.7123, 4.7906) (21.7235, 4.7969) (21.7348, 4.8033) (21.7462, 4.8097) (21.7576, 4.8161) (21.769, 4.8226) (21.7805, 4.8292) (21.792, 4.8358) (21.8035, 4.8425) (21.8151, 4.8492) (21.8267, 4.8559) (21.8384, 4.8628) (21.8501, 4.8696) (21.8618, 4.8765) (21.8736, 4.8835) (21.8854, 4.8905) (21.8972, 4.8976) (21.9091, 4.9048) (21.921, 4.9119) (21.9329, 4.9192) (21.9449, 4.9265) (21.9569, 4.9338) (21.9689, 4.9412) (21.981, 4.9486) (21.9931, 4.9561) (22.0052, 4.9637) (22.0174, 4.9713) (22.0296, 4.9789) (22.0418, 4.9866) (22.0541, 4.9944) (22.0663, 5.0022) (22.0786, 5.01) (22.091, 5.018) (22.1034, 5.0259) (22.1158, 5.0339) (22.1282, 5.042) (22.1406, 5.0501) (22.1531, 5.0583) (22.1656, 5.0665) (22.1782, 5.0748) (22.1907, 5.0831) (22.2033, 5.0915) (22.216, 5.0999) (22.2286, 5.1084) (22.2413, 5.1169) (22.254, 5.1255) (22.2667, 5.1341) (22.2794, 5.1428) (22.2922, 5.1516) (22.305, 5.1603) (22.3178, 5.1692) (22.3307, 5.1781) (22.3435, 5.187) (22.3564, 5.196) (22.3693, 5.2051) (22.3823, 5.2142) (22.3952, 5.2233) (22.4082, 5.2325) (22.4212, 5.2418) (22.4342, 5.2511) (22.4473, 5.2604) (22.4603, 5.2698) (22.4734, 5.2793) (22.4865, 5.2888) (22.4996, 5.2983) (22.5128, 5.3079) (22.526, 5.3176) (22.5391, 5.3273) (22.5524, 5.3371) (22.5656, 5.3469) (22.5788, 5.3568) (22.5921, 5.3667) (22.6054, 5.3766) (22.6187, 5.3867) (22.632, 5.3967) (22.6453, 5.4068) (22.6587, 5.417) (22.672, 5.4272) (22.6854, 5.4375) (22.6988, 5.4478) (22.7122, 5.4582) (22.7257, 5.4686) (22.7391, 5.4791) (22.7526, 5.4896) (22.7661, 5.5002) (22.7795, 5.5108) (22.7931, 5.5215) (22.8066, 5.5322) (22.8201, 5.543) (22.8337, 5.5538) (22.8473, 5.5647) (22.8608, 5.5756) (22.8744, 5.5866) (22.888, 5.5976) (22.9017, 5.6087) (22.9153, 5.6198) (22.929, 5.631) (22.9426, 5.6422) (22.9563, 5.6535) (22.97, 5.6648) (22.9837, 5.6762) (22.9974, 5.6876) (23.0111, 5.6991) (23.0248, 5.7106) (23.0386, 5.7222) (23.0523, 5.7338) (23.0661, 5.7455) (23.0799, 5.7572) (23.0937, 5.769) (23.1075, 5.7808) (23.1213, 5.7927) (23.1351, 5.8046) (23.1489, 5.8166) (23.1628, 5.8286) (23.1766, 5.8407) (23.1905, 5.8528) (23.2043, 5.865) (23.2182, 5.8772) (23.2321, 5.8895) (23.2432, 5.8993) (23.2516, 5.9067) (23.2571, 5.9117) (23.2599, 5.9142) knots 0 0 0 0 0 0 0.00416667 0.00833333 0.0125 0.01666667 0.02083333 0.025 0.02916667 0.03333333 0.0375 0.04166667 0.04583333 0.05 0.05416667 0.05833333 0.0625 0.06666667 0.07083333 0.075 0.07916667 0.08333333 0.0875 0.09166667 0.09583333 0.1 0.10416667 0.10833333 0.1125 0.11666667 0.12083333 0.125 0.12916667 0.13333333 0.1375 0.14166667 0.14583333 0.15 0.15416667 0.15833333 0.1625 0.16666667 0.17083333 0.175 0.17916667 0.18333333 0.1875 0.19166667 0.19583333 0.2 0.20416667 0.20833333 0.2125 0.21666667 0.22083333 0.225 0.22916667 0.23333333 0.2375 0.24166667 0.24583333 0.25 0.25416667 0.25833333 0.2625 0.26666667 0.27083333 0.275 0.27916667 0.28333333 0.2875 0.29166667 0.29583333 0.3 0.30416667 0.30833333 0.3125 0.31666667 0.32083333 0.325 0.32916667 0.33333333 0.3375 0.34166667 0.34583333 0.35 0.35416667 0.35833333 0.3625 0.36666667 0.37083333 0.375 0.37916667 0.38333333 0.3875 0.39166667 0.39583333 0.4 0.40416667 0.40833333 0.4125 0.41666667 0.42083333 0.425 0.42916667 0.43333333 0.4375 0.44166667 0.44583333 0.45 0.45416667 0.45833333 0.4625 0.46666667 0.47083333 0.475 0.47916667 0.48333333 0.4875 0.49166667 0.49583333 0.5 0.50416667 0.50833333 0.5125 0.51666667 0.52083333 0.525 0.52916667 0.53333333 0.5375 0.54166667 0.54583333 0.55 0.55416667 0.55833333 0.5625 0.56666667 0.57083333 0.575 0.57916667 0.58333333 0.5875 0.59166667 0.59583333 0.6 0.60416667 0.60833333 0.6125 0.61666667 0.62083333 0.625 0.62916667 0.63333333 0.6375 0.64166667 0.64583333 0.65 0.65416667 0.65833333 0.6625 0.66666667 0.67083333 0.675 0.67916667 0.68333333 0.6875 0.69166667 0.69583333 0.7 0.70416667 0.70833333 0.7125 0.71666667 0.72083333 0.725 0.72916667 0.73333333 0.7375 0.74166667 0.74583333 0.75 0.75416667 0.75833333 0.7625 0.76666667 0.77083333 0.775 0.77916667 0.78333333 0.7875 0.79166667 0.79583333 0.8 0.80416667 0.80833333 0.8125 0.81666667 0.82083333 0.825 0.82916667 0.83333333 0.8375 0.84166667 0.84583333 0.85 0.85416667 0.85833333 0.8625 0.86666667 0.87083333 0.875 0.87916667 0.88333333 0.8875 0.89166667 0.89583333 0.9 0.90416667 0.90833333 0.9125 0.91666667 0.92083333 0.925 0.92916667 0.93333333 0.9375 0.94166667 0.94583333 0.95 0.95416667 0.95833333 0.9625 0.96666667 0.97083333 0.975 0.97916667 0.98333333 0.9875 0.99166667 0.99583333 1 1 1 1 1 1
  arc A3 (23.2599, 5.9142) -> (22.7649, 7.5999) centre (0, 0) ccw
  spline S3 degree 5 poles (22.7649, 7.5999) (22.7612, 7.6005) (22.7539, 7.6017) (22.7428, 7.6034) (22.7282, 7.6057) (22.7099, 7.6085) (22.6916, 7.6113) (22.6733, 7.614) (22.6551, 7.6167) (22.637, 7.6194) (22.6188, 7.622) (22.6007, 7.6246) (22.5826, 7.6272) (22.5646, 7.6297) (22.5466, 7.6322) (22.5286, 7.6347) (22.5107, 7.6371) (22.4928, 7.6394) (22.4749, 7.6418) (22.4571, 7.6441) (22.4393, 7.6464) (22.4216, 7.6486) (22.4039, 7.6508) (22.3862, 7.653) (22.3686, 7.6551) (22.351, 7.6572) (22.3334, 7.6592) (22.3159, 7.6613) (22.2984, 7.6632) (22.2809, 7.6652) (22.2635, 7.6671) (22.2462, 7.669) (22.2288, 7.6708) (22.2115, 7.6727) (22.1943, 7.6744) (22.1771, 7.6762) (22.1599, 7.6779) (22.1427, 7.6796) (22.1256, 7.6812) (22.1086, 7.6828) (22.0916, 7.6844) (22.0746, 7.6859) (22.0577, 7.6874) (22.0408, 7.6889) (22.0239, 7.6903) (22.0071, 7.6917) (21.9903, 7.6931) (21.9736, 7.6945) (21.9569, 7.6958) (21.9403, 7.697) (21.9237, 7.6983) (21.9071, 7.6995) (21.8906, 7.7006) (21.8741, 7.7018) (21.8577, 7.7029) (21.8413, 7.704) (21.825, 7.705) (21.8087, 7.706) (21.7924, 7.707) (21.7762, 7.7079) (21.76, 7.7088) (21.7439, 7.7097) (21.7278, 7.7106) (21.7118, 7.7114) (21.6958, 7.7122) (21.6799, 7.7129) (21.664, 7.7136) (21.6481, 7.7143) (21.6323, 7.715) (21.6166, 7.7156) (21.6009, 7.7162) (21.5852, 7.7168) (21.5696, 7.7173) (21.5541, 7.7178) (21.5385, 7.7183) (21.5231, 7.7188) (21.5077, 7.7192) (21.4923, 7.7196) (21.477, 7.7199) (21.4617, 7.7202) (21.4465, 7.7205) (21.4313, 7.7208) (21.4162, 7.721) (21.4011, 7.7213) (21.3861, 7.7214) (21.3711, 7.7216) (21.3562, 7.7217) (21.3413, 7.7218) (21.3265, 7.7219) (21.3117, 7.7219) (21.297, 7.7219) (21.2824, 7.7219) (21.2678, 7.7219) (21.2532, 7.7218) (21.2387, 7.7217) (21.2243, 7.7216) (21.2099, 7.7214) (21.1955, 7.7212) (21.1812, 7.721) (21.167, 7.7208) (21.1528, 7.7205) (21.1387, 7.7202) (21.1247, 7.7199) (21.1106, 7.7196) (21.0967, 7.7192) (21.0828, 7.7188) (21.069, 7.7184) (21.0552, 7.7179) (21.0415, 7.7175) (21.0278, 7.717) (21.0142, 7.7165) (21.0006, 7.7159) (20.9871, 7.7154) (20.9737, 7.7148) (20.9603, 7.7141) (20.947, 7.7135) (20.9338, 7.7128) (20.9206, 7.7122) (20.9074, 7.7115) (20.8944, 7.7107) (20.8814, 7.71) (20.8684, 7.7092) (20.8555, 7.7084) (20.8427, 7.7076) (20.8299, 7.7067) (20.8172, 7.7059) (20.8046, 7.705) (20.792, 7.7041) (20.7795, 7.7031) (20.7671, 7.7022) (20.7547, 7.7012) (20.7424, 7.7002) (20.7302, 7.6992) (20.718, 7.6982) (20.7059, 7.6971) (20.6938, 7.6961) (20.6819, 7.695) (20.6699, 7.6939) (20.6581, 7.6927) (20.6463, 7.6916) (20.6346, 7.6904) (20.623, 7.6893) (20.6114, 7.6881) (20.5999, 7.6868) (20.5885, 7.6856) (20.5771, 7.6844) (20.5659, 7.6831) (20.5547, 7.6818) (20.5435, 7.6805) (20.5325, 7.6792) (20.5215, 7.6779) (20.5105, 7.6765) (20.4997, 7.6752) (20.4889, 7.6738) (20.4782, 7.6724) (20.4676, 7.671) (20.4571, 7.6696) (20.4466, 7.6682) (20.4362, 7.6668) (20.4259, 7.6653) (20.4157, 7.6639) (20.4055, 7.6624) (20.3955, 7.6609) (20.3855, 7.6594) (20.3756, 7.6579) (20.3657, 7.6564) (20.356, 7.6549) (20.3463, 7.6533) (20.3367, 7.6518) (20.3272, 7.6502) (20.3178, 7.6487) (20.3085, 7.6471) (20.2992, 7.6455) (20.2901, 7.644) (20.281, 7.6424) (20.272, 7.6408) (20.2631, 7.6392) (20.2543, 7.6376) (20.2456, 7.636) (20.2369, 7.6343) (20.2284, 7.6327) (20.2199, 7.6311) (20.2116, 7.6295) (20.2033, 7.6279) (20.1951, 7.6262) (20.1871, 7.6246) (20.1791, 7.623) (20.1712, 7.6213) (20.1634, 7.6197) (20.1557, 7.6181) (20.1481, 7.6165) (20.1406, 7.6148) (20.1332, 7.6132) (20.1259, 7.6116) (20.1187, 7.61) (20.1116, 7.6084) (20.1046, 7.6068) (20.0977, 7.6052) (20.0909, 7.6036) (20.0843, 7.602) (20.0777, 7.6004) (20.0712, 7.5989) (20.0649, 7.5973) (20.0586, 7.5958) (20.0525, 7.5942) (20.0465, 7.5927) (20.0406, 7.5912) (20.0348, 7.5897) (20.0291, 7.5882) (20.0235, 7.5868) (20.0181, 7.5853) (20.0128, 7.5839) (20.0076, 7.5825) (20.0025, 7.5811) (19.9975, 7.5797) (19.9927, 7.5783) (19.988, 7.577) (19.9834, 7.5757) (19.979, 7.5744) (19.9747, 7.5731) (19.9705, 7.5719) (19.9664, 7.5707) (19.9625, 7.5695) (19.9587, 7.5684) (19.9551, 7.5673) (19.9516, 7.5662) (19.9482, 7.5651) (19.945, 7.5641) (19.942, 7.5631) (19.9391, 7.5622) (19.9363, 7.5613) (19.9337, 7.5604) (19.9312, 7.5596) (19.9289, 7.5588) (19.9268, 7.5581) (19.9248, 7.5574) (19.923, 7.5568) (19.9214, 7.5563) (19.9199, 7.5557) (19.9186, 7.5553) (19.9175, 7.5549) (19.9168, 7.5546) (19.9163, 7.5544) (19.916, 7.5543) (19.9159, 7.5543) knots -1 -1 -1 -1 -1 -1 -0.99583333 -0.99166667 -0.9875 -0.98333333 -0.97916667 -0.975 -0.97083333 -0.96666667 -0.9625 -0.95833333 -0.95416667 -0.95 -0.94583333 -0.94166667 -0.9375 -0.93333333 -0.92916667 -0.925 -0.92083333 -0.91666667 -0.9125 -0.90833333 -0.90416667 -0.9 -0.89583333 -0.89166667 -0.8875 -0.88333333 -0.87916667 -0.875 -0.87083333 -0.86666667 -0.8625 -0.85833333 -0.85416667 -0.85 -0.84583333 -0.84166667 -0.8375 -0.83333333 -0.82916667 -0.825 -0.82083333 -0.81666667 -0.8125 -0.80833333 -0.80416667 -0.8 -0.79583333 -0.79166667 -0.7875 -0.78333333 -0.77916667 -0.775 -0.77083333 -0.76666667 -0.7625 -0.75833333 -0.75416667 -0.75 -0.74583333 -0.74166667 -0.7375 -0.73333333 -0.72916667 -0.725 -0.72083333 -0.71666667 -0.7125 -0.70833333 -0.70416667 -0.7 -0.69583333 -0.69166667 -0.6875 -0.68333333 -0.67916667 -0.675 -0.67083333 -0.66666667 -0.6625 -0.65833333 -0.65416667 -0.65 -0.64583333 -0.64166667 -0.6375 -0.63333333 -0.62916667 -0.625 -0.62083333 -0.61666667 -0.6125 -0.60833333 -0.60416667 -0.6 -0.59583333 -0.59166667 -0.5875 -0.58333333 -0.57916667 -0.575 -0.57083333 -0.56666667 -0.5625 -0.55833333 -0.55416667 -0.55 -0.54583333 -0.54166667 -0.5375 -0.53333333 -0.52916667 -0.525 -0.52083333 -0.51666667 -0.5125 -0.50833333 -0.50416667 -0.5 -0.49583333 -0.49166667 -0.4875 -0.48333333 -0.47916667 -0.475 -0.47083333 -0.46666667 -0.4625 -0.45833333 -0.45416667 -0.45 -0.44583333 -0.44166667 -0.4375 -0.43333333 -0.42916667 -0.425 -0.42083333 -0.41666667 -0.4125 -0.40833333 -0.40416667 -0.4 -0.39583333 -0.39166667 -0.3875 -0.38333333 -0.37916667 -0.375 -0.37083333 -0.36666667 -0.3625 -0.35833333 -0.35416667 -0.35 -0.34583333 -0.34166667 -0.3375 -0.33333333 -0.32916667 -0.325 -0.32083333 -0.31666667 -0.3125 -0.30833333 -0.30416667 -0.3 -0.29583333 -0.29166667 -0.2875 -0.28333333 -0.27916667 -0.275 -0.27083333 -0.26666667 -0.2625 -0.25833333 -0.25416667 -0.25 -0.24583333 -0.24166667 -0.2375 -0.23333333 -0.22916667 -0.225 -0.22083333 -0.21666667 -0.2125 -0.20833333 -0.20416667 -0.2 -0.19583333 -0.19166667 -0.1875 -0.18333333 -0.17916667 -0.175 -0.17083333 -0.16666667 -0.1625 -0.15833333 -0.15416667 -0.15 -0.14583333 -0.14166667 -0.1375 -0.13333333 -0.12916667 -0.125 -0.12083333 -0.11666667 -0.1125 -0.10833333 -0.10416667 -0.1 -0.09583333 -0.09166667 -0.0875 -0.08333333 -0.07916667 -0.075 -0.07083333 -0.06666667 -0.0625 -0.05833333 -0.05416667 -0.05 -0.04583333 -0.04166667 -0.0375 -0.03333333 -0.02916667 -0.025 -0.02083333 -0.01666667 -0.0125 -0.00833333 -0.00416667 0 0 0 0 0 0
  line L6 (19.9159, 7.5543) -> (19.9147, 7.5539)
  line L7 (19.9147, 7.5539) -> (18.2325, 6.9158)
  arc A4 (18.2325, 6.9158) -> (17.1663, 9.2503) centre (0, 0) ccw
  line L8 (17.1663, 9.2503) -> (18.7502, 10.1038)
  line L9 (18.7502, 10.1038) -> (18.7513, 10.1044)